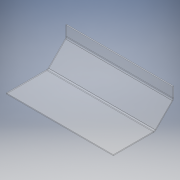
# Autodesk Inventor part: 10mm Polycarb
Saved by Autodesk Inventor 2018 (Build 220112000, 112)
## iProperties
Created: 2018-09-18
Part Number: 10mm Polycarb
Material: Polycarbonate, Clear
Document SubType Name: Sheet Metal
Designer: P301319
Density: 1.2 g/cm^3
Sheet Metal Rule: Polycarb 10mm
Appearance: Polycarbonate - Clear
Author: P301319
Autodesk Inventor part; units mm, degrees
ref_plane "YZ Plane" through (0, 0, 0) normal (1, 0, 0) x (0, 1, 0)
ref_plane "XZ Plane" through (0, 0, 0) normal (0, 1, 0) x (-1, 0, 0)
ref_plane "XY Plane" through (0, 0, 0) normal (0, 0, 1) x (1, 0, 0)
sketch "Sketch1" plane through (0, 0, 0) normal (0, 0, 1) x (1, 0, 0)
  line L0 (0, 0) -> (1100, 0)
  line L1 (1100, 0) -> (1100, 430)
  line L2 (1100, 430) -> (0, 430)
  line L3 (0, 430) -> (0, 0)
  dimension "d0" = 1100
  dimension "d1" = 430
  measures "d0" distance of L2.end L1.end
  measures "d1" distance of L1.end L0.end
extrude "Plate1" add sketch "Sketch1" along normal blind 10
sketch "Sketch2" plane through (0, 422.9289, 7.0711) normal (0, 0.7071068, -0.7071068) x (-1, 0, 0)
  line L0 (-1100, 0) -> (0, 0)
  line L1 (0, 0) -> (0, 270)
  line L2 (0, 270) -> (-1100, 270)
  line L3 (-1100, 270) -> (-1100, 0)
  constraints: 6 end point, 1 horizontal, 1 perpendicular, 1 vertical
edge flange "Flange1" height 270 angle 45 thickness 10 bend radius 20 thickness toward (0, 0.7071068, -0.7071068) relief straight relief width 10 relief depth 5 edges at (550, 430, 10) wall of the first edge with corners at (1100, 422.9289, 7.0711) (0, 422.9289, 7.0711) (0, 613.8478, 197.9899) (1100, 613.8478, 197.9899)
bend "Bend1"
corner "Corner1"
sketch "Sketch3" plane through (0, 610.9188, 190.9188) normal (0, 1, 0) x (-1, 0, 0)
  line L0 (-1100, 0) -> (0, 0)
  line L1 (0, 0) -> (0, 120)
  line L2 (0, 120) -> (-1100, 120)
  line L3 (-1100, 120) -> (-1100, 0)
  constraints: 6 end point, 1 horizontal, 1 perpendicular, 1 vertical
edge flange "Flange2" height 120 angle 45 thickness 10 bend radius 20 thickness toward (0, 1, 0) relief straight relief width 10 relief depth 5 edges at (550, 613.8478, 197.9899) wall of the first edge with corners at (1100, 610.9188, 190.9188) (0, 610.9188, 190.9188) (0, 610.9188, 310.9188) (1100, 610.9188, 310.9188)
bend "Bend2"
corner "Corner2"
equation "\"d2\" = Thickness"
equation "\"d3\" = BendReliefWidth"
equation "\"d4\" = BendReliefDepth"
equation "\"d5\" = MinimumRemnant"
equation "\"d6\" = TransitionRadius"
equation "\"d10\" = CornerReliefSize"
equation "\"d11\" = GapSize"
equation "\"d12\" = JacobiRadiusSize"
equation "\"d13\" = BendReliefWidth"
equation "\"d14\" = BendReliefDepth"
equation "\"d15\" = MinimumRemnant"
equation "\"d16\" = TransitionRadius"
equation "\"d20\" = CornerReliefSize"
equation "\"d21\" = GapSize"
equation "\"d22\" = JacobiRadiusSize"
equation "\"BendReliefDepth\" = 0.5 * Thickness"
equation "\"Thickness\" = 10"
equation "\"BendReliefWidth\" = 10"
equation "\"MinimumRemnant\" = 20"
equation "\"TransitionRadius\" = 10"
equation "\"CornerReliefSize\" = 40"
equation "\"GapSize\" = 10"
equation "\"JacobiRadiusSize\" = 10"
body "Solid1"
